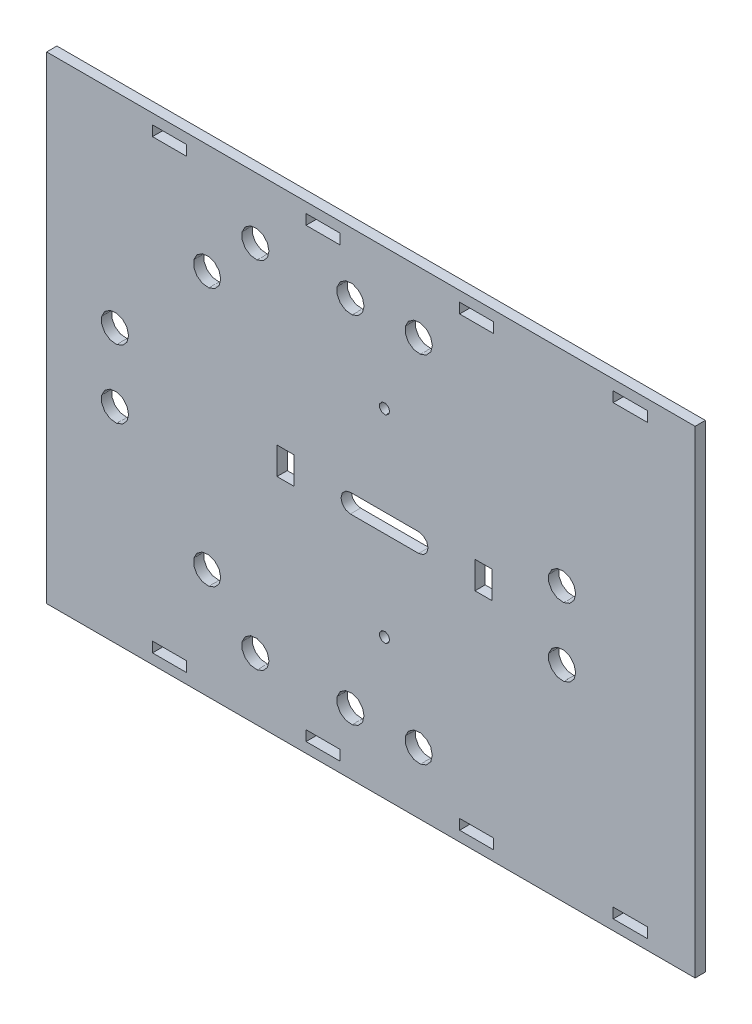
# Autodesk Inventor part: top_plate
Saved by Autodesk Inventor 2019.3 (Build 233278000, 278)
## iProperties
Created: 2019-03-22
Part Number: top_plate
Material: Generic
Document SubType Name: Modeling
Designer: Dave
Density: 1 g/cm^3
Appearance: Default
Author: Dave
Autodesk Inventor part; units mm, degrees
ref_plane "YZ Plane" through (0, 0, 0) normal (1, 0, 0) x (0, 1, 0)
ref_plane "XZ Plane" through (0, 0, 0) normal (0, 1, 0) x (-1, 0, 0)
ref_plane "XY Plane" through (0, 0, 0) normal (0, 0, 1) x (1, 0, 0)
sketch "Sketch1" plane through (0, 0, 0) normal (0, 0, 1) x (1, 0, 0)
  line L0 (0, 0) -> (190, 0)
  line L1 (190, 0) -> (190, 140)
  line L2 (190, 140) -> (0, 140)
  line L3 (0, 140) -> (0, 0)
  circle A0 centre (89, 122) radius 4
  line L4 (73, 110) -> (125, 110) construction
  line L5 (125, 110) -> (125, 30) construction
  line L6 (125, 30) -> (73, 30) construction
  line L7 (73, 30) -> (73, 110) construction
  line L8 (59, 96) -> (139, 96) construction
  line L9 (139, 96) -> (139, 44) construction
  line L10 (139, 44) -> (59, 44) construction
  line L11 (59, 44) -> (59, 96) construction
  line L12 (32, 85) -> (59, 85) construction
  line L13 (59, 85) -> (59, 55) construction
  line L14 (59, 55) -> (32, 55) construction
  line L15 (32, 55) -> (32, 85) construction
  circle A1 centre (99, 122) radius 4 construction
  circle A2 centre (109, 122) radius 4
  circle A3 centre (151, 79.9878) radius 4
  circle A4 centre (151, 69.9878) radius 4 construction
  circle A5 centre (151, 59.9878) radius 4
  circle A6 centre (109, 18) radius 4
  circle A7 centre (99, 18) radius 4 construction
  circle A8 centre (89, 18) radius 4
  circle A9 centre (20, 79.9878) radius 4
  circle A10 centre (20, 69.9878) radius 4 construction
  circle A11 centre (20, 59.9878) radius 4
  circle A12 centre (61.1421, 122) radius 4
  circle A13 centre (54.0711, 114.9289) radius 4 construction
  circle A14 centre (54.0711, 25.0711) radius 4 construction
  circle A15 centre (61.1421, 18) radius 4
  line L16 (61.1421, 122) -> (54.0711, 114.9289) construction
  line L17 (54.0711, 25.0711) -> (61.1421, 18) construction
  line L18 (73, 110) -> (59, 96) construction
  circle A16 centre (47, 107.8579) radius 4
  circle A17 centre (47, 32.1421) radius 4
  line L19 (47, 107.8579) -> (54.0711, 114.9289) construction
  line L20 (47, 32.1421) -> (54.0711, 25.0711) construction
  line L21 (54.0711, 114.9289) -> (66, 103) construction
  line L22 (59, 44) -> (73, 30) construction
  line L23 (66, 37) -> (54.0711, 25.0711) construction
  line L24 (31, 137) -> (41, 137)
  line L25 (41, 137) -> (41, 134)
  line L26 (41, 134) -> (31, 134)
  line L27 (31, 134) -> (31, 137)
  line L28 (76, 137) -> (86, 137)
  line L29 (86, 137) -> (86, 134)
  line L30 (86, 134) -> (76, 134)
  line L31 (76, 134) -> (76, 137)
  line L32 (121, 137) -> (131, 137)
  line L33 (131, 137) -> (131, 134)
  line L34 (131, 134) -> (121, 134)
  line L35 (121, 134) -> (121, 137)
  line L36 (166, 137) -> (176, 137)
  line L37 (176, 137) -> (176, 134)
  line L38 (176, 134) -> (166, 134)
  line L39 (166, 134) -> (166, 137)
  line L40 (31, 6) -> (41, 6)
  line L41 (41, 6) -> (41, 3)
  line L42 (41, 3) -> (31, 3)
  line L43 (31, 3) -> (31, 6)
  line L44 (76, 6) -> (86, 6)
  line L45 (86, 6) -> (86, 3)
  line L46 (86, 3) -> (76, 3)
  line L47 (76, 3) -> (76, 6)
  line L48 (121, 6) -> (131, 6)
  line L49 (131, 6) -> (131, 3)
  line L50 (131, 3) -> (121, 3)
  line L51 (121, 3) -> (121, 6)
  line L52 (166, 6) -> (176, 6)
  line L53 (176, 6) -> (176, 3)
  line L54 (176, 3) -> (166, 3)
  line L55 (166, 3) -> (166, 6)
  line L56 (89, 70) -> (109, 70) construction
  line L57 (89, 67.25) -> (109, 67.25)
  line L58 (109, 72.75) -> (89, 72.75)
  arc A18 (89, 72.75) -> (89, 67.25) centre (89, 70) ccw
  arc A19 (109, 67.25) -> (109, 72.75) centre (109, 70) ccw
  circle A20 centre (99, 99) radius 1.5
  circle A21 centre (99, 41) radius 1.5
  line L59 (130.5, 66) -> (125.5, 66)
  line L60 (125.5, 66) -> (125.5, 74)
  line L61 (125.5, 74) -> (130.5, 74)
  line L62 (130.5, 74) -> (130.5, 66)
  line L63 (72.5, 66) -> (67.5, 66)
  line L64 (67.5, 66) -> (67.5, 74)
  line L65 (67.5, 74) -> (72.5, 74)
  line L66 (72.5, 74) -> (72.5, 66)
  point P0 (95, 140)
  point P1 (190, 70)
  point P2 (99, 110)
  point P3 (99, 96)
  point P4 (59, 70)
  point P5 (32, 70)
  point P6 (99, 70)
  point P7 (59, 70)
  point P8 (128, 66)
  point P9 (70, 66)
  point P10 (125.5, 70)
  point P11 (72.5, 70)
  dimension "d3" = 8
  dimension "d5" = 140
  dimension "d6" = 190
  dimension "d7" = 80
  dimension "d8" = 52
  dimension "d9" = 80
  dimension "d10" = 52
  dimension "d11" = 27
  dimension "d12" = 30
  dimension "d13" = 10
  dimension "d14" = 10
  dimension "d15" = 10
  dimension "d16" = 10
  dimension "d17" = 12
  dimension "d18" = 12
  dimension "d19" = 12
  dimension "d20" = 12
  dimension "d21" = 10
  dimension "d35" = 10
  dimension "d36" = 3
  dimension "d38" = 45
  dimension "d39" = 45
  dimension "d40" = 45
  dimension "d41" = 24
  dimension "d42" = 3
  dimension "d43" = 3
  dimension "d46" = 5.5
  dimension "d47" = 20
  dimension "d48" = 3
  dimension "d49" = 29
  dimension "d50" = 29
  dimension "d54" = 73.9878
  dimension "d56" = 91
  dimension "d60" = 5
  dimension "d61" = 29
  dimension "d62" = 29
  dimension "d63" = 8
  constraints: 136 end point, 32 parallel, 22 centre point, 21 point on line, 17 equal radius, 16 perpendicular, 15 horizontal, 14 midpoint, 13 horizontal alignment, 12 vertical alignment, 10 equal length, 4 point on circle, 4 tangent, 2 collinear
  measures "d3" diameter of A0
  measures "d5" distance of L0.end L1.end
  measures "d6" distance of L1.end L2.end
  measures "d7" distance of L4.end L5.end
  measures "d8" distance of L4.start L4.end
  measures "d9" distance of L8.start L8.end
  measures "d10" distance of L10.end L8.start
  measures "d11" distance of L12.start L12.end
  measures "d12" distance of L14.end L12.start
  measures "d13" distance of A1.centre A0.centre
  measures "d14" distance of A2.centre A1.centre
  measures "d15" distance of A10.centre A9.centre
  measures "d16" distance of A11.centre A10.centre
  measures "d17" distance of point (99, 110) A1.centre
  measures "d18" distance from line of L9 A3.centre
  measures "d19" distance from line of L15 A9.centre
  measures "d20" distance from line of L6 A7.centre
  measures "d21" distance of L16.start L16.end
  measures "d35" distance of L25.end L26.end
  measures "d36" distance of L24.end L25.end
  measures "d38" distance between parallel lines of L33 L37
  measures "d39" distance between parallel lines of L29 L33
  measures "d40" distance between parallel lines of L25 L29
  measures "d41" distance between parallel lines of L1 L39
  measures "d42" distance between parallel lines of L2 L24
  measures "d43" distance between parallel lines of L0 L54
  measures "d46" distance between parallel lines of L58 L57
  measures "d47" distance from line of L3 A9.centre
  measures "d48" diameter of A20
  measures "d49" distance of A21.centre point (99, 70)
  measures "d50" distance of point (99, 70) A20.centre
  measures "d54" distance from line of A3.centre L52
  measures "d56" distance from line of A20.centre L1
  measures "d60" distance of L59.start L59.end
  measures "d61" horizontal distance of point (99, 70) point (128, 66)
  measures "d62" horizontal distance of point (99, 70) point (70, 66)
  measures "d63" distance of L61.end L59.start
extrude "Extrusion4" add sketch "Sketch1" along normal blind 3
body "Solid4"
